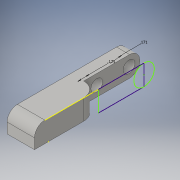
# Autodesk Inventor part: fire-bar
Saved by Autodesk Inventor 2016 SP1 (Build 200210100, 210)
## iProperties
Created: 2016-05-01
Part Number: fire-bar
Material: Generic
Document SubType Name: Modeling
Designer: Wes
Density: 1 g/cm^3
Appearance: Default
Author: Wes
Autodesk Inventor part; units mm, degrees
ref_plane "YZ Plane" through (0, 0, 0) normal (1, 0, 0) x (0, 1, 0)
ref_plane "XZ Plane" through (0, 0, 0) normal (0, 1, 0) x (-1, 0, 0)
ref_plane "XY Plane" through (0, 0, 0) normal (0, 0, 1) x (1, 0, 0)
sketch "Block1" plane through (0, 0, 0) normal (0, 0, 1) x (1, 0, 0)
  circle A0 centre (40.64, 3.81) radius 3.81
  point P0 (32.0567, 3.81)
sketch "Sketch1" plane through (0, 0, 0) normal (0, 1, 0) x (-1, 0, 0)
  line L0 (5.08, 5.08) -> (-5.08, 5.08)
  line L1 (-5.08, 5.08) -> (-5.08, -39.37)
  line L2 (-5.08, -39.37) -> (5.08, -39.37)
  line L3 (5.08, -39.37) -> (5.08, 5.08)
  point P0 (0, 0)
  dimension "d0" = 10.16
  dimension "d1" = 44.45
  constraints: 8 end point, 2 parallel, 1 horizontal, 1 perpendicular
  measures "d0" distance of L2.end L1.end
  measures "d1" distance of L1.end L0.end
extrude "bar" add sketch "Sketch1" along normal blind 7.62
sketch "Sketch2" plane through (-5.08, 0, -39.37) normal (-1, 0, 0) x (0, 0, 1)
  circle A0 centre (4, 3.81) radius 2.175
  circle A1 centre (16, 3.81) radius 2.175
  circle A2 centre (9.9822, 3.81) radius 1.0704
  point P0 (39.37, 0)
  dimension "d4" = 4.35
  dimension "d5" = 4.35
  constraints: 3 centre point
  measures "d4" diameter of A0
  measures "d5" diameter of A1
hole "pegholes" at (-5.08, 3.81, -35.37) at (-5.08, 3.81, -23.37) direction (1, 0, 0) diameter 4.35 end through all
fillet "Fillet3" radius 3.81 3 edges at (0, 7.62, -39.37) (0, 0, -39.37) (0, 7.62, 5.08)
sketch "Sketch3" plane through (5.08, 0, 5.08) normal (1, 0, 0) x (0, 0, -1)
  line L0 (40.64, 7.62) -> (3.81, 7.62) projected
  line L1 (23.6161, 7.62) -> (40.64, 7.62)
  line L2 (40.64, 7.62) -> (40.64, 0)
  line L3 (40.64, 0) -> (23.6161, 0)
  line L4 (23.6161, 0) -> (23.6161, 7.62)
  circle A0 centre (40.64, 3.81) radius 3.81
  point P0 (5.08, 0)
  constraints: 8 end point, 2 parallel, 1 horizontal, 1 perpendicular, 1 point on line
extrude "Extrusion2" cut sketch "Sketch3" against normal blind 5.334 contours A0 L2 | L2 A0
extrude "Extrusion3" cut sketch "Sketch3" against normal blind 5.334 contours A0 L3 L4 L0 | L2 A0 picked at (39.3793, 3.6569)
fillet "Fillet4" radius 5.334 1 edges at (5.08, 3.81, -18.5361)
body "Solid1"
